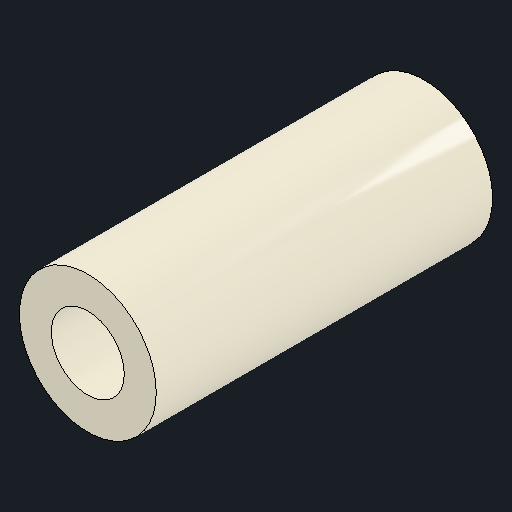
# Autodesk Inventor part: ignition-alumina-tube-upper
Saved by Autodesk Inventor 2027.1 (Build 311270010, 270A)
## iProperties
Created: 2026-10-02
Part Number: ignition-alumina-tube-upper
Material: Alumina
Description: Alumina ignition clamp tube; provisional OD 6 mm, bore 3.2 mm, length 14.750000 mm; extends to holding nut facing surface. Physical properties require verification.
Document SubType Name: Modeling
Designer: queezz
Density: 1 g/cm^3
Appearance: Alumina ivory
Mass: 0.178585 g
Surface Area: 2.95586 cm^2
Volume: 0.178585 cm^3
Author: queezz
Autodesk Inventor part; units mm, degrees
ref_plane "YZ Plane" through (0, 0, 0) normal (1, 0, 0) x (0, 1, 0)
ref_plane "XZ Plane" through (0, 0, 0) normal (0, 1, 0) x (-1, 0, 0)
ref_plane "XY Plane" through (0, 0, 0) normal (0, 0, 1) x (1, 0, 0)
sketch "Tube OD 6 mm - bore 3.2 mm" plane through (0, 0, 0) normal (0, 0, 1) x (1, 0, 0)
  circle A0 centre (0, 0) radius 3
  circle A1 centre (0, 0) radius 1.6
  dimension "d0" = 14.75
  constraints: 2 centre point
extrude "Tube length" add sketch "Tube OD 6 mm - bore 3.2 mm" along normal blind 14.75
body "Solid1"
